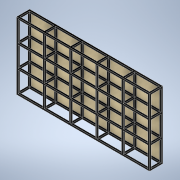
# Autodesk Inventor part: CustomAquariumsStand
Saved by Autodesk Inventor 2022 (Build 260153000, 153)
## iProperties
Created: 2021-06-25
Part Number: CustomAquariumsStand
Material: Generic
Document SubType Name: Modeling
Designer: jamieson-bl
Density: 1 g/cm^3
Appearance: Default
Author: jamieson-bl
Autodesk Inventor part; units mm, degrees
ref_plane "YZ Plane" through (0, 0, 0) normal (1, 0, 0) x (0, 1, 0)
ref_plane "XZ Plane" through (0, 0, 0) normal (0, 1, 0) x (-1, 0, 0)
ref_plane "XY Plane" through (0, 0, 0) normal (0, 0, 1) x (1, 0, 0)
sketch "Sketch1" plane through (0, 0, 0) normal (0, 0, 1) x (1, 0, 0)
  line L0 (1524, -762) -> (-1524, -762)
  line L1 (-1524, -762) -> (-1524, 762)
  line L2 (-1524, 762) -> (1524, 762)
  line L3 (1524, 762) -> (1524, -762)
  line L4 (1524, -762) -> (-1524, 762) construction
  line L5 (-1524, -762) -> (1524, 762) construction
  point P0 (0, 0)
  dimension "d0" = 3048
  dimension "d1" = 1524
  constraints: 12 end point, 2 midpoint, 2 parallel, 1 horizontal, 1 perpendicular
  measures "d0" distance of L1.end L2.end
  measures "d1" distance of L0.end L1.end
extrude "Extrusion1" add sketch "Sketch1" along normal blind 19.05
sketch "Sketch2" plane through (0, 0, 19.05) normal (0, 0, 1) x (1, 0, 0)
  line L0 (-1543.05, -781.05) -> (1543.05, -781.05)
  line L1 (1543.05, -781.05) -> (1543.05, 781.05)
  line L2 (1543.05, 781.05) -> (-1543.05, 781.05)
  line L3 (-1543.05, 781.05) -> (-1543.05, -781.05)
  line L4 (-1543.05, -781.05) -> (1543.05, 781.05) construction
  line L5 (1543.05, -781.05) -> (-1543.05, 781.05) construction
  line L6 (1504.95, -742.95) -> (-1504.95, -742.95)
  line L7 (-1504.95, -742.95) -> (-1504.95, 742.95)
  line L8 (-1504.95, 742.95) -> (1504.95, 742.95)
  line L9 (1504.95, 742.95) -> (1504.95, -742.95)
  line L10 (1504.95, -742.95) -> (-1504.95, 742.95) construction
  line L11 (-1504.95, -742.95) -> (1504.95, 742.95) construction
  point P0 (0, 0)
  dimension "d4" = 3086.1
  dimension "d5" = 1562.1
  dimension "d6" = 3009.9
  dimension "d7" = 1485.9
  constraints: 24 end point, 4 midpoint, 4 parallel, 2 horizontal, 2 perpendicular
  measures "d4" distance of L2.end L1.end
  measures "d5" distance of L1.end L0.end
  measures "d6" distance of L7.end L8.end
  measures "d7" distance of L6.end L7.end
extrude "Extrusion2" add sketch "Sketch2" along normal blind 38.1
sketch "Sketch4" plane through (0, 0, 19.05) normal (0, 0, 1) x (1, 0, 0)
  line L0 (-1504.95, 742.95) -> (-1504.95, -742.95) projected
  line L1 (-1543.05, 781.05) -> (-1504.95, 781.05)
  line L2 (-1504.95, 781.05) -> (-1504.95, 742.95)
  line L3 (-1504.95, 742.95) -> (-1543.05, 742.95)
  line L4 (-1543.05, 742.95) -> (-1543.05, 781.05)
  line L5 (-1504.95, 234.95) -> (-1543.05, 234.95)
  line L6 (-1504.95, 273.05) -> (-1504.95, 234.95)
  line L7 (-1543.05, 273.05) -> (-1504.95, 273.05)
  line L8 (-1543.05, 234.95) -> (-1543.05, 273.05)
  line L9 (-1504.95, -273.05) -> (-1543.05, -273.05)
  line L10 (-1504.95, -234.95) -> (-1504.95, -273.05)
  line L11 (-1543.05, -234.95) -> (-1504.95, -234.95)
  line L12 (-1543.05, -273.05) -> (-1543.05, -234.95)
  line L13 (-1504.95, -781.05) -> (-1543.05, -781.05)
  line L14 (-1504.95, -742.95) -> (-1504.95, -781.05)
  line L15 (-1543.05, -742.95) -> (-1504.95, -742.95)
  line L16 (-1543.05, -781.05) -> (-1543.05, -742.95)
  line L17 (-895.35, 742.95) -> (-933.45, 742.95)
  line L18 (-895.35, 781.05) -> (-895.35, 742.95)
  line L19 (-933.45, 781.05) -> (-895.35, 781.05)
  line L20 (-933.45, 742.95) -> (-933.45, 781.05)
  line L21 (-895.35, 234.95) -> (-933.45, 234.95)
  line L22 (-895.35, 273.05) -> (-895.35, 234.95)
  line L23 (-933.45, 273.05) -> (-895.35, 273.05)
  line L24 (-933.45, 234.95) -> (-933.45, 273.05)
  line L25 (-895.35, -273.05) -> (-933.45, -273.05)
  line L26 (-895.35, -234.95) -> (-895.35, -273.05)
  line L27 (-933.45, -234.95) -> (-895.35, -234.95)
  line L28 (-933.45, -273.05) -> (-933.45, -234.95)
  line L29 (-895.35, -781.05) -> (-933.45, -781.05)
  line L30 (-895.35, -742.95) -> (-895.35, -781.05)
  line L31 (-933.45, -742.95) -> (-895.35, -742.95)
  line L32 (-933.45, -781.05) -> (-933.45, -742.95)
  line L33 (-285.75, 742.95) -> (-323.85, 742.95)
  line L34 (-285.75, 781.05) -> (-285.75, 742.95)
  line L35 (-323.85, 781.05) -> (-285.75, 781.05)
  line L36 (-323.85, 742.95) -> (-323.85, 781.05)
  line L37 (-285.75, 234.95) -> (-323.85, 234.95)
  line L38 (-285.75, 273.05) -> (-285.75, 234.95)
  line L39 (-323.85, 273.05) -> (-285.75, 273.05)
  line L40 (-323.85, 234.95) -> (-323.85, 273.05)
  line L41 (-285.75, -273.05) -> (-323.85, -273.05)
  line L42 (-285.75, -234.95) -> (-285.75, -273.05)
  line L43 (-323.85, -234.95) -> (-285.75, -234.95)
  line L44 (-323.85, -273.05) -> (-323.85, -234.95)
  line L45 (-285.75, -781.05) -> (-323.85, -781.05)
  line L46 (-285.75, -742.95) -> (-285.75, -781.05)
  line L47 (-323.85, -742.95) -> (-285.75, -742.95)
  line L48 (-323.85, -781.05) -> (-323.85, -742.95)
  line L49 (323.85, 742.95) -> (285.75, 742.95)
  line L50 (323.85, 781.05) -> (323.85, 742.95)
  line L51 (285.75, 781.05) -> (323.85, 781.05)
  line L52 (285.75, 742.95) -> (285.75, 781.05)
  line L53 (323.85, 234.95) -> (285.75, 234.95)
  line L54 (323.85, 273.05) -> (323.85, 234.95)
  line L55 (285.75, 273.05) -> (323.85, 273.05)
  line L56 (285.75, 234.95) -> (285.75, 273.05)
  line L57 (323.85, -273.05) -> (285.75, -273.05)
  line L58 (323.85, -234.95) -> (323.85, -273.05)
  line L59 (285.75, -234.95) -> (323.85, -234.95)
  line L60 (285.75, -273.05) -> (285.75, -234.95)
  line L61 (323.85, -781.05) -> (285.75, -781.05)
  line L62 (323.85, -742.95) -> (323.85, -781.05)
  line L63 (285.75, -742.95) -> (323.85, -742.95)
  line L64 (285.75, -781.05) -> (285.75, -742.95)
  line L65 (933.45, 742.95) -> (895.35, 742.95)
  line L66 (933.45, 781.05) -> (933.45, 742.95)
  line L67 (895.35, 781.05) -> (933.45, 781.05)
  line L68 (895.35, 742.95) -> (895.35, 781.05)
  line L69 (933.45, 234.95) -> (895.35, 234.95)
  line L70 (933.45, 273.05) -> (933.45, 234.95)
  line L71 (895.35, 273.05) -> (933.45, 273.05)
  line L72 (895.35, 234.95) -> (895.35, 273.05)
  line L73 (933.45, -273.05) -> (895.35, -273.05)
  line L74 (933.45, -234.95) -> (933.45, -273.05)
  line L75 (895.35, -234.95) -> (933.45, -234.95)
  line L76 (895.35, -273.05) -> (895.35, -234.95)
  line L77 (933.45, -781.05) -> (895.35, -781.05)
  line L78 (933.45, -742.95) -> (933.45, -781.05)
  line L79 (895.35, -742.95) -> (933.45, -742.95)
  line L80 (895.35, -781.05) -> (895.35, -742.95)
  line L81 (1543.05, 742.95) -> (1504.95, 742.95)
  line L82 (1543.05, 781.05) -> (1543.05, 742.95)
  line L83 (1504.95, 781.05) -> (1543.05, 781.05)
  line L84 (1504.95, 742.95) -> (1504.95, 781.05)
  line L85 (1543.05, 234.95) -> (1504.95, 234.95)
  line L86 (1543.05, 273.05) -> (1543.05, 234.95)
  line L87 (1504.95, 273.05) -> (1543.05, 273.05)
  line L88 (1504.95, 234.95) -> (1504.95, 273.05)
  line L89 (1543.05, -273.05) -> (1504.95, -273.05)
  line L90 (1543.05, -234.95) -> (1543.05, -273.05)
  line L91 (1504.95, -234.95) -> (1543.05, -234.95)
  line L92 (1504.95, -273.05) -> (1504.95, -234.95)
  line L93 (1543.05, -781.05) -> (1504.95, -781.05)
  line L94 (1543.05, -742.95) -> (1543.05, -781.05)
  line L95 (1504.95, -742.95) -> (1543.05, -742.95)
  line L96 (1504.95, -781.05) -> (1504.95, -742.95)
  point P0 (0, 0)
  dimension "d12" = 508
  dimension "d15" = 609.6
  constraints: 192 end point, 2 horizontal, 2 parallel, 1 collinear, 1 perpendicular, 1 vertical, 183 other
  measures "d12" distance of L0.start L5.start
  measures "d15" distance of L0.start L17.start
extrude "Extrusion3" add sketch "Sketch4" along normal blind 304.8
sketch "Sketch5" plane through (0, 0, 19.05) normal (0, 0, 1) x (1, 0, 0)
  line L0 (-1504.95, 273.05) -> (-1543.05, 273.05) projected
  line L1 (-895.35, 234.95) -> (-933.45, 234.95) projected
  line L2 (-1504.95, 273.05) -> (-933.45, 273.05)
  line L3 (-933.45, 273.05) -> (-933.45, 234.95)
  line L4 (-933.45, 234.95) -> (-1504.95, 234.95)
  line L5 (-1504.95, 234.95) -> (-1504.95, 273.05)
  line L6 (1504.95, 742.95) -> (-1504.95, 742.95) projected
  line L7 (-895.35, 273.05) -> (-895.35, 234.95) projected
  line L8 (-933.45, 742.95) -> (-895.35, 742.95)
  line L9 (-895.35, 742.95) -> (-895.35, 273.05)
  line L10 (-895.35, 273.05) -> (-933.45, 273.05)
  line L11 (-933.45, 273.05) -> (-933.45, 742.95)
  line L12 (-1504.95, -273.05) -> (-1504.95, -234.95)
  line L13 (-1504.95, -234.95) -> (-933.45, -234.95)
  line L14 (-933.45, -273.05) -> (-1504.95, -273.05)
  line L15 (-933.45, -234.95) -> (-933.45, 234.95)
  line L16 (-895.35, 234.95) -> (-895.35, -234.95)
  line L17 (-933.45, -234.95) -> (-933.45, -273.05)
  line L18 (-895.35, -234.95) -> (-933.45, -234.95)
  line L19 (-933.45, 234.95) -> (-895.35, 234.95)
  line L20 (-1504.95, -781.05) -> (-1504.95, -742.95)
  line L21 (-1504.95, -742.95) -> (-933.45, -742.95)
  line L22 (-933.45, -781.05) -> (-1504.95, -781.05)
  line L23 (-933.45, -742.95) -> (-933.45, -273.05)
  line L24 (-895.35, -273.05) -> (-895.35, -742.95)
  line L25 (-933.45, -742.95) -> (-933.45, -781.05)
  line L26 (-895.35, -742.95) -> (-933.45, -742.95)
  line L27 (-933.45, -273.05) -> (-895.35, -273.05)
  line L28 (-895.35, 234.95) -> (-895.35, 273.05)
  line L29 (-895.35, 273.05) -> (-323.85, 273.05)
  line L30 (-323.85, 234.95) -> (-895.35, 234.95)
  line L31 (-323.85, 273.05) -> (-323.85, 742.95)
  line L32 (-285.75, 742.95) -> (-285.75, 273.05)
  line L33 (-323.85, 273.05) -> (-323.85, 234.95)
  line L34 (-285.75, 273.05) -> (-323.85, 273.05)
  line L35 (-323.85, 742.95) -> (-285.75, 742.95)
  line L36 (-895.35, -273.05) -> (-895.35, -234.95)
  line L37 (-895.35, -234.95) -> (-323.85, -234.95)
  line L38 (-323.85, -273.05) -> (-895.35, -273.05)
  line L39 (-323.85, -234.95) -> (-323.85, 234.95)
  line L40 (-285.75, 234.95) -> (-285.75, -234.95)
  line L41 (-323.85, -234.95) -> (-323.85, -273.05)
  line L42 (-285.75, -234.95) -> (-323.85, -234.95)
  line L43 (-323.85, 234.95) -> (-285.75, 234.95)
  line L44 (-895.35, -781.05) -> (-895.35, -742.95)
  line L45 (-895.35, -742.95) -> (-323.85, -742.95)
  line L46 (-323.85, -781.05) -> (-895.35, -781.05)
  line L47 (-323.85, -742.95) -> (-323.85, -273.05)
  line L48 (-285.75, -273.05) -> (-285.75, -742.95)
  line L49 (-323.85, -742.95) -> (-323.85, -781.05)
  line L50 (-285.75, -742.95) -> (-323.85, -742.95)
  line L51 (-323.85, -273.05) -> (-285.75, -273.05)
  line L52 (-285.75, 234.95) -> (-285.75, 273.05)
  line L53 (-285.75, 273.05) -> (285.75, 273.05)
  line L54 (285.75, 234.95) -> (-285.75, 234.95)
  line L55 (285.75, 273.05) -> (285.75, 742.95)
  line L56 (323.85, 742.95) -> (323.85, 273.05)
  line L57 (285.75, 273.05) -> (285.75, 234.95)
  line L58 (323.85, 273.05) -> (285.75, 273.05)
  line L59 (285.75, 742.95) -> (323.85, 742.95)
  line L60 (-285.75, -273.05) -> (-285.75, -234.95)
  line L61 (-285.75, -234.95) -> (285.75, -234.95)
  line L62 (285.75, -273.05) -> (-285.75, -273.05)
  line L63 (285.75, -234.95) -> (285.75, 234.95)
  line L64 (323.85, 234.95) -> (323.85, -234.95)
  line L65 (285.75, -234.95) -> (285.75, -273.05)
  line L66 (323.85, -234.95) -> (285.75, -234.95)
  line L67 (285.75, 234.95) -> (323.85, 234.95)
  line L68 (-285.75, -781.05) -> (-285.75, -742.95)
  line L69 (-285.75, -742.95) -> (285.75, -742.95)
  line L70 (285.75, -781.05) -> (-285.75, -781.05)
  line L71 (285.75, -742.95) -> (285.75, -273.05)
  line L72 (323.85, -273.05) -> (323.85, -742.95)
  line L73 (285.75, -742.95) -> (285.75, -781.05)
  line L74 (323.85, -742.95) -> (285.75, -742.95)
  line L75 (285.75, -273.05) -> (323.85, -273.05)
  line L76 (323.85, 234.95) -> (323.85, 273.05)
  line L77 (323.85, 273.05) -> (895.35, 273.05)
  line L78 (895.35, 234.95) -> (323.85, 234.95)
  line L79 (895.35, 273.05) -> (895.35, 742.95)
  line L80 (933.45, 742.95) -> (933.45, 273.05)
  line L81 (895.35, 273.05) -> (895.35, 234.95)
  line L82 (933.45, 273.05) -> (895.35, 273.05)
  line L83 (895.35, 742.95) -> (933.45, 742.95)
  line L84 (323.85, -273.05) -> (323.85, -234.95)
  line L85 (323.85, -234.95) -> (895.35, -234.95)
  line L86 (895.35, -273.05) -> (323.85, -273.05)
  line L87 (895.35, -234.95) -> (895.35, 234.95)
  line L88 (933.45, 234.95) -> (933.45, -234.95)
  line L89 (895.35, -234.95) -> (895.35, -273.05)
  line L90 (933.45, -234.95) -> (895.35, -234.95)
  line L91 (895.35, 234.95) -> (933.45, 234.95)
  line L92 (323.85, -781.05) -> (323.85, -742.95)
  line L93 (323.85, -742.95) -> (895.35, -742.95)
  line L94 (895.35, -781.05) -> (323.85, -781.05)
  line L95 (895.35, -742.95) -> (895.35, -273.05)
  line L96 (933.45, -273.05) -> (933.45, -742.95)
  line L97 (895.35, -742.95) -> (895.35, -781.05)
  line L98 (933.45, -742.95) -> (895.35, -742.95)
  line L99 (895.35, -273.05) -> (933.45, -273.05)
  line L100 (933.45, 234.95) -> (933.45, 273.05)
  line L101 (933.45, 273.05) -> (1504.95, 273.05)
  line L102 (1504.95, 234.95) -> (933.45, 234.95)
  line L103 (1504.95, 273.05) -> (1504.95, 742.95)
  line L104 (1543.05, 742.95) -> (1543.05, 273.05)
  line L105 (1504.95, 273.05) -> (1504.95, 234.95)
  line L106 (1543.05, 273.05) -> (1504.95, 273.05)
  line L107 (1504.95, 742.95) -> (1543.05, 742.95)
  line L108 (933.45, -273.05) -> (933.45, -234.95)
  line L109 (933.45, -234.95) -> (1504.95, -234.95)
  line L110 (1504.95, -273.05) -> (933.45, -273.05)
  line L111 (1504.95, -234.95) -> (1504.95, 234.95)
  line L112 (1543.05, 234.95) -> (1543.05, -234.95)
  line L113 (1504.95, -234.95) -> (1504.95, -273.05)
  line L114 (1543.05, -234.95) -> (1504.95, -234.95)
  line L115 (1504.95, 234.95) -> (1543.05, 234.95)
  line L116 (933.45, -781.05) -> (933.45, -742.95)
  line L117 (933.45, -742.95) -> (1504.95, -742.95)
  line L118 (1504.95, -781.05) -> (933.45, -781.05)
  line L119 (1504.95, -742.95) -> (1504.95, -273.05)
  line L120 (1543.05, -273.05) -> (1543.05, -742.95)
  line L121 (1504.95, -742.95) -> (1504.95, -781.05)
  line L122 (1543.05, -742.95) -> (1504.95, -742.95)
  line L123 (1504.95, -273.05) -> (1543.05, -273.05)
  point P0 (0, 0)
  dimension "d22" = 508
  dimension "d25" = 609.6
  constraints: 240 end point, 16 point on line, 4 parallel, 3 horizontal, 2 collinear, 2 perpendicular, 1 vertical, 222 other
  measures "d22" distance of L4.end L12.start
  measures "d25" distance of L4.end L28.start
extrude "Extrusion4" add sketch "Sketch5" along normal blind 38.1 contours L16 L18 L15 L1 | L7 L29 L33 L30 | L4 L5 L2 L3 | L10 L11 L6 L9 | L37 L41 L38 L36 | L43 L40 L42 L39 | L17 L14 L12 L13 | L31 L6 L32 L34 | L24 L26 L23 L27 | L52 L53 L57 L54 | L51 L48 L50 L47 | L61 L65 L62 L60 | L67 L64 L66 L63 | L55 L6 L56 L58 | L76 L77 L81 L78 | L75 L72 L74 L71 | L85 L89 L86 L84 | L91 L88 L90 L87 | L79 L6 L80 L82 | L100 L101 L105 L102 | L99 L96 L98 L95 | L109 L113 L110 L108
pattern_linear "Rectangular Pattern1" count 2 spacing 266.7 along (0, 0, 1) of "Extrusion4", "Extrusion2"
body "Solid1"
